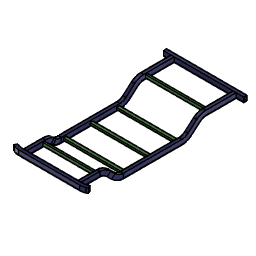
Chassis CAD Model (Autodesk Fusion 360 design; units mm, degrees)
Autodesk Fusion 360 part; units mm, degrees
sketch "Sketch1" plane through (0, 0, 0) normal (0, 0, 1) x (1, 0, 0)
  line L0 (-88.2341, -43) -> (1522.2341, -43)
  line L1 (-206.7424, -18.6008) -> (-250, 0)
  line L2 (1640.7424, -18.6008) -> (1684, 0)
  arc A0 (1522.2341, -43) -> (1640.7424, -18.6008) centre (1522.2341, 257) ccw
  arc A1 (-206.7424, -18.6008) -> (-88.2341, -43) centre (-88.2341, 257) ccw
  point P0 (0, -43)
  constraint tangent L0 A0
  constraint tangent L2 A0
  constraint tangent L0 A1
  constraint tangent L1 A1
sketch "Sketch2" plane through (0, 0, 0) normal (1, 0, 0) x (0, 0, -1)
  line L0 (0, 0) -> (0, 493.2962)
  line L1 (84.3286, 708.3443, -33.7314) -> (165.6714, 793.5607, -66.2686)
  line L2 (250, 1008.6088, -100) -> (250, 2556.9675, -100)
  line L3 (175.7938, 2754.4951, -100) -> (-25.7938, 2984.9299, -100)
  line L4 (-100, 3182.4575, -100) -> (-100, 3979.755, -100)
  arc A0 through (84.3286, 708.3443, -33.7314) (21.9468, 610.0168, -8.7787) (0, 493.2962, 0)
  arc A1 through (250, 1008.6088, -100) (228.0532, 891.8882, -91.2213) (165.6714, 793.5607, -66.2686)
  arc A2 through (250, 2556.9675, -100) (230.8364, 2662.4707, -100) (175.7938, 2754.4951, -100)
  arc A3 through (-100, 3182.4575, -100) (-80.8364, 3076.9543, -100) (-25.7938, 2984.9299, -100)
  line L5 (-56.9, -7.5) -> (56.9, -7.5)
  line L6 (56.9, -7.5) -> (56.9, -78.5)
  line L7 (56.9, -78.5) -> (-56.9, -78.5)
  line L8 (-56.9, -78.5) -> (-56.9, -7.5)
  line L9 (-64.5, 0) -> (64.5, 0)
  line L10 (64.5, 0) -> (64.5, -86)
  line L11 (64.5, -86) -> (-64.5, -86)
  line L12 (-64.5, -86) -> (-64.5, 0)
sketch "Sketch3" plane through (0, 0, 0) normal (0, 1, 0) x (1, 0, 0)
  line L0 (35.4, 56.9) -> (-35.4, 56.9)
  line L1 (-35.4, 56.9) -> (-35.4, -56.9)
  line L2 (-35.4, -56.9) -> (35.4, -56.9)
  line L3 (35.4, -56.9) -> (35.4, 56.9)
  line L4 (43, 64.5) -> (-43, 64.5)
  line L5 (-43, 64.5) -> (-43, -64.5)
  line L6 (-43, -64.5) -> (43, -64.5)
  line L7 (43, -64.5) -> (43, 64.5)
sweep "Sweep1" add profiles "Sketch3" path "Sketch2" along L0 A0 L1 A1 L2 A2 L3 A3 L4 section 1 makes body 1
ref_plane "WorkPlane1" through (717, 246.6481, 0) normal (1, 0, 0) x (0, 0, -1)
mirror "Mirror1" about plane through (717, 246.6481, 0) normal (1, 0, 0) of bodies 1 makes body 2
ref_plane "WorkPlane2" through (43, 0, 0) normal (1, 0, 0) x (0, 1, 0)
sketch "Sketch4" plane through (43, 0, 0) normal (1, 0, 0) x (0, 0, -1)
  line L0 (36, 472.5) -> (-36, 472.5)
  line L1 (-36, 472.5) -> (-36, 427.5)
  line L2 (-36, 427.5) -> (36, 427.5)
  line L3 (36, 427.5) -> (36, 472.5)
  line L4 (41, 477.5) -> (-41, 477.5)
  line L5 (-41, 477.5) -> (-41, 422.5)
  line L6 (-41, 422.5) -> (41, 422.5)
  line L7 (41, 422.5) -> (41, 477.5)
ref_plane "WorkPlane3" through (-57, 0, 0) normal (1, 0, 0) x (0, 1, 0)
sketch "Sketch5" plane through (-57, 0, 0) normal (1, 0, 0) x (0, 0, -1)
  line L0 (275, 1135.955) -> (230, 1135.955)
  line L1 (230, 1135.955) -> (230, 1063.955)
  line L2 (230, 1063.955) -> (275, 1063.955)
  line L3 (275, 1063.955) -> (275, 1135.955)
  line L4 (280, 1140.955) -> (225, 1140.955)
  line L5 (225, 1140.955) -> (225, 1058.955)
  line L6 (225, 1058.955) -> (280, 1058.955)
  line L7 (280, 1058.955) -> (280, 1140.955)
  line L8 (275, 1835.92) -> (230, 1835.92)
  line L9 (230, 1835.92) -> (230, 1763.92)
  line L10 (230, 1763.92) -> (275, 1763.92)
  line L11 (275, 1763.92) -> (275, 1835.92)
  line L12 (280, 1840.92) -> (225, 1840.92)
  line L13 (225, 1840.92) -> (225, 1758.92)
  line L14 (225, 1758.92) -> (280, 1758.92)
  line L15 (280, 1758.92) -> (280, 1840.92)
  line L16 (275, 2535.885) -> (230, 2535.885)
  line L17 (230, 2535.885) -> (230, 2463.885)
  line L18 (230, 2463.885) -> (275, 2463.885)
  line L19 (275, 2463.885) -> (275, 2535.885)
  line L20 (280, 2540.885) -> (225, 2540.885)
  line L21 (225, 2540.885) -> (225, 2458.885)
  line L22 (225, 2458.885) -> (280, 2458.885)
  line L23 (280, 2458.885) -> (280, 2540.885)
  line L24 (-136, 3272.255) -> (-64, 3272.255)
  line L25 (-64, 3272.255) -> (-64, 3227.255)
  line L26 (-64, 3227.255) -> (-136, 3227.255)
  line L27 (-136, 3227.255) -> (-136, 3272.255)
  line L28 (-141, 3277.255) -> (-59, 3277.255)
  line L29 (-59, 3277.255) -> (-59, 3222.255)
  line L30 (-59, 3222.255) -> (-141, 3222.255)
  line L31 (-141, 3222.255) -> (-141, 3277.255)
extrude "Extrude1" add sketch "Sketch5" sketch "Sketch4" along normal up to near side of body 2 separate body of sketch 2 makes body 3 at (459, 3277.255, 113.6667) makes body 4 at (459, 1086.2883, -280) makes body 5 at (459, 1786.2533, -280) makes body 6 at (459, 2486.2183, -280) makes body 7 at (492.3333, 477.5, -13.6667)
ref_plane "WorkPlane4" through (-343, 0, 0) normal (1, 0, 0) x (0, 1, 0)
sketch "Sketch6" plane through (-343, 0, 0) normal (1, 0, 0) x (0, 0, -1)
  line L0 (-156.9, 4058.155) -> (-43.1, 4058.155)
  line L1 (-43.1, 4058.155) -> (-43.1, 3987.355)
  line L2 (-43.1, 3987.355) -> (-156.9, 3987.355)
  line L3 (-156.9, 3987.355) -> (-156.9, 4058.155)
  line L4 (-164.5, 4065.755) -> (-35.5, 4065.755)
  line L5 (-35.5, 4065.755) -> (-35.5, 3979.755)
  line L6 (-35.5, 3979.755) -> (-164.5, 3979.755)
  line L7 (-164.5, 3979.755) -> (-164.5, 4065.755)
extrude "Extrude2" add sketch "Sketch6" along normal blind 2120 separate body makes body 8
sweep "Sweep2" add profiles "Sketch2" path "Sketch1" along L2 A0 L0 A1 L1 section 1 separate body makes body 9
